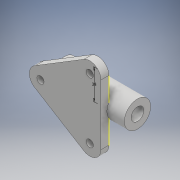
# Autodesk Inventor part: Figure 5.37
Saved by Autodesk Inventor 2018 (Build 220112000, 112)
## iProperties
Created: 2018-01-25
Part Number: Figure 5.37
Material: Generic
Document SubType Name: Modeling
Designer: udyll
Density: 1 g/cm^3
Appearance: Default
Author: udyll
Autodesk Inventor part; units mm, degrees
ref_plane "YZ Plane" through (0, 0, 0) normal (1, 0, 0) x (0, 1, 0)
ref_plane "XZ Plane" through (0, 0, 0) normal (0, 1, 0) x (-1, 0, 0)
ref_plane "XY Plane" through (0, 0, 0) normal (0, 0, 1) x (1, 0, 0)
sketch "Sketch1" plane through (0, 0, 0) normal (0, 1, 0) x (-1, 0, 0)
  arc A0 (9.8478, 9.9509) -> (-14, 0) centre (0, 0) ccw
  line L0 (0, 0) -> (76, 0) construction
  line L1 (0, -76) -> (61.9125, -76) construction
  arc A1 (66.3277, -51.1998) -> (68.0769, -25.2732) centre (62, -37.8855) ccw
  arc A2 (68.2906, -50.3927) -> (68.2245, -25.3454) centre (62, -37.8855) ccw
  arc A3 (7.3403, 11.9214) -> (-14, 0) centre (0, 0) ccw
  arc A4 (-14, -76) -> (7.3403, -87.9214) centre (0, -76) ccw
  line L2 (70.3359, -49.1333) -> (7.3403, -87.9214)
  line L3 (70.3359, -26.6378) -> (7.3403, 11.9214)
  line L4 (-14, 0) -> (-14, -76)
  arc A5 (-14, -76) -> (7.3403, -87.9214) centre (0, -76) ccw
  point P0 (4.6474, 13.2061)
  point P1 (4.7589, -89.1664)
  dimension "d37" = 62
  dimension "d40" = 76
  dimension "d41" = 62
  constraints: 16 point on circle, 10 end point, 6 centre point, 4 coincident, 2 horizontal, 2 point on line, 2 tangent, 1 vertical
  measures "d37" horizontal distance of point (0, 0) A1.centre
  measures "d40" distance of L1.start point (0, 0)
  measures "d41" horizontal distance of L1.start A1.centre
extrude "Extrusion1" add sketch "Sketch1" against normal blind 10 contours L3 A1 L2 A4 L4 A0 | A1 L3
sketch "Sketch2" plane through (0, -10, 0) normal (0, -1, 0) x (1, 0, 0)
  circle A0 centre (0, 0) radius 4.5
  arc A1 (-7.3403, -87.9214) -> (14, -76) centre (0, -76) ccw projected
  circle A2 centre (0, -76) radius 4.5
  arc A3 (-68.2245, -25.3454) -> (-70.3359, -49.1333) centre (-62, -37.8855) ccw projected
  circle A4 centre (-62, -37.8855) radius 4.5
  dimension "d10" = 9
  dimension "d42" = 9
  dimension "d43" = 9
  dimension "d44" = 62
  constraints: 3 centre point, 3 coincident
  measures "d10" diameter of A0
  measures "d42" diameter of A2
  measures "d43" diameter of A4
  measures "d44" horizontal distance of A2.centre A4.centre
extrude "Extrusion2" cut sketch "Sketch2" against normal blind 10
sketch "Sketch8" plane through (0, 0, 0) normal (0, 1, 0) x (1, 0, 0)
  line L0 (0, 0) -> (0, 38)
  line L1 (0, 38) -> (14, 38)
  line L2 (14, 76) -> (14, 0) projected
  dimension "d45" = 38
  constraints: 4 end point, 1 midpoint, 1 vertical
  measures "d45" distance of L0.start L0.end
sketch "Sketch9" plane through (14, 0, 0) normal (1, 0, 0) x (0, 0, -1)
  line L0 (76, -10) -> (0, -10) projected
  line L1 (38, -10) -> (38, 14)
  circle A0 centre (38, 14) radius 16.5
  point P0 (0, 0)
  dimension "d46" = 24
  dimension "d47" = 33
  constraints: 2 end point, 1 centre point, 1 coincident, 1 midpoint, 1 vertical
  measures "d46" distance of L1.start L1.end
  measures "d47" diameter of A0
extrude "Extrusion6" add sketch "Sketch9" against normal blind 70
sketch "Sketch10" plane through (14, -10, 0) normal (1, 0, 0) x (0, 0, -1)
  arc A0 (46.7321, 10) -> (29.2679, 10) centre (38, 24) ccw projected
  circle A1 centre (38, 24) radius 16.5
  point P0 (0, 10)
  constraints: 1 centre point, 1 coincident
extrude "Extrusion7" add sketch "Sketch10" along normal blind 22
sketch "Sketch11" plane through (36, 14, -38) normal (1, 0, 0) x (0, 0, -1)
  circle A0 centre (0, 0) radius 8
  point P0 (-38, -14)
  dimension "d52" = 16
  constraints: 1 centre point
  measures "d52" diameter of A0
extrude "Extrusion8" cut sketch "Sketch11" against normal blind 70
body "Solid1"
